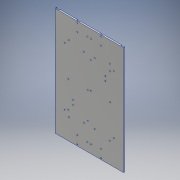
# Autodesk Inventor part: 밑판_수정
Saved by Autodesk Inventor 2017 (Build 210142000, 142)
## iProperties
Part Number: 밑판_수정
Material: 알루미늄 6061
Document SubType Name: Modeling
Designer: minom
Density: 2.7 g/cm^3
Appearance: 알루미늄 - 평지
Mass: 247.223 g
Surface Area: 1507.76 cm^2
Volume: 91.564 cm^3
Author: minom
Autodesk Inventor part; units mm, degrees
(part 1 of 2)
ref_plane "YZ Plane" through (0, 0, 0) normal (1, 0, 0) x (0, 1, 0)
ref_plane "XZ Plane" through (0, 0, 0) normal (0, 1, 0) x (-1, 0, 0)
ref_plane "XY Plane" through (0, 0, 0) normal (0, 0, 1) x (1, 0, 0)
sketch "스케치1" plane through (0, 0, 0) normal (0, 1, 0) x (-1, 0, 0)
  line L0 (0, 0) -> (-190, 0)
  line L1 (-190, 0) -> (-190, 300)
  line L2 (-190, 300) -> (0, 300)
  line L3 (0, 260) -> (0, 40)
  line L4 (0, 0) -> (40, 0)
  line L5 (40, 0) -> (40, 40)
  line L6 (40, 40) -> (0, 40)
  line L7 (0, 40) -> (0, 0)
  line L8 (-190, 0) -> (-230, 0)
  line L9 (-230, 0) -> (-230, 40)
  line L10 (-230, 40) -> (-190, 40)
  line L11 (-190, 40) -> (-190, 0)
  line L12 (-190, 300) -> (-230, 300)
  line L13 (-230, 300) -> (-230, 260)
  line L14 (-230, 260) -> (-190, 260)
  line L15 (-190, 260) -> (-190, 300)
  line L16 (0, 300) -> (40, 300)
  line L17 (40, 300) -> (40, 260)
  line L18 (40, 260) -> (0, 260)
  line L19 (0, 260) -> (0, 300)
  dimension "d0" = 190
  dimension "d1" = 300
  dimension "d2" = 40
  dimension "d3" = 40
  dimension "d4" = 40
  dimension "d5" = 40
  dimension "d6" = 40
  dimension "d7" = 40
  dimension "d8" = 40
  dimension "d9" = 40
  constraints: 40 end point, 10 parallel, 5 horizontal, 5 perpendicular
  measures "d0" distance of L1.end L2.end
  measures "d1" distance of L0.end L1.end
  measures "d2" distance of L3.end L5.end
  measures "d3" distance of L5.end L4.end
  measures "d4" distance of L9.end L10.end
  measures "d5" distance of L8.end L9.end
  measures "d6" distance of L14.end L13.end
  measures "d7" distance of L13.end L12.end
  measures "d8" distance of L3.start L17.end
  measures "d9" distance of L16.end L17.end
extrude "돌출1" add sketch "스케치1" along normal blind 4
sketch "스케치2" plane through (0, 4, 0) normal (0, 1, 0) x (1, 0, 0)
  line L0 (230, 0) -> (-40, 0) projected
  line L1 (-40, 0) -> (-40, -40) projected
  line L2 (-40, -40) -> (0, -40) projected
  line L3 (0, -40) -> (0, -260) projected
  line L4 (0, -260) -> (-40, -260) projected
  line L5 (-40, -260) -> (-40, -300) projected
  line L6 (-40, -300) -> (230, -300) projected
  line L7 (230, -300) -> (230, -260) projected
  line L8 (230, -260) -> (190, -260) projected
  line L9 (190, -260) -> (190, -40) projected
  line L10 (190, -40) -> (230, -40) projected
  line L11 (230, -40) -> (230, 0) projected
  line L12 (230, 0) -> (-40, 0) projected
  line L13 (-39, 0) -> (-30.8, 0)
  line L14 (-30.8, 0) -> (-30.8, -40)
  line L15 (-30.8, -40) -> (-39, -40)
  line L16 (-39, -40) -> (-39, 0)
  line L17 (-40, -300) -> (230, -300) projected
  line L18 (1, 0) -> (9.2, 0)
  line L19 (9.2, 0) -> (9.2, -300)
  line L20 (9.2, -300) -> (1, -300)
  line L21 (1, -300) -> (1, 0)
  line L22 (0, -260) -> (-40, -260) projected
  line L23 (-39, -260) -> (-30.8, -260)
  line L24 (-30.8, -260) -> (-30.8, -300)
  line L25 (-30.8, -300) -> (-39, -300)
  line L26 (-39, -300) -> (-39, -260)
  line L27 (190, -40) -> (230, -40) projected
  line L28 (229, 0) -> (220.8, 0)
  line L29 (220.8, 0) -> (220.8, -40)
  line L30 (220.8, -40) -> (229, -40)
  line L31 (229, -40) -> (229, 0)
  line L32 (189, 0) -> (180.8, 0)
  line L33 (180.8, 0) -> (180.8, -300)
  line L34 (180.8, -300) -> (189, -300)
  line L35 (189, -300) -> (189, 0)
  line L36 (229, -260) -> (220.8, -260)
  line L37 (220.8, -260) -> (220.8, -300)
  line L38 (220.8, -300) -> (229, -300)
  line L39 (229, -300) -> (229, -260)
  point P0 (0, 0)
  dimension "d12" = 8.2
  dimension "d13" = 8.2
  dimension "d14" = 8.2
  dimension "d15" = 8.2
  dimension "d16" = 1
  dimension "d17" = 1
  dimension "d18" = 1
  dimension "d19" = 1
  constraints: 48 end point, 16 point on line, 12 parallel, 6 horizontal, 6 perpendicular
  measures "d12" distance of L14.end L15.end
  measures "d13" distance of L19.end L20.end
  measures "d14" distance of L30.end L29.end
  measures "d15" distance of L34.end L33.end
  measures "d16" distance between parallel lines of L26 L5
  measures "d17" distance between parallel lines of L21 L3
  measures "d18" distance between parallel lines of L11 L31
  measures "d19" distance between parallel lines of L35 L9
extrude "돌출2" cut sketch "스케치2" against normal blind 2 contours L31 L10 L29 L0 | L35 L6 L33 L0 | L19 L6 L21 L0 | L37 L8 L39 L6 | L14 L2 L16 L0 | L6 L26 L4 L24
sketch "스케치4" plane through (0, 0, 0) normal (0, -1, 0) x (1, 0, 0)
  line L0 (220.8, 300) -> (220.8, 260) projected
  line L1 (220.8, 260) -> (190, 260) projected
  line L2 (190, 260) -> (190, 40) projected
  line L3 (190, 40) -> (220.8, 40) projected
  line L4 (220.8, 40) -> (220.8, 0) projected
  line L5 (220.8, 0) -> (189, 0) projected
  line L6 (189, 0) -> (189, 300) projected
  line L7 (189, 300) -> (220.8, 300) projected
  line L8 (9.2, 0) -> (9.2, 300) projected
  line L9 (9.2, 300) -> (180.8, 300) projected
  line L10 (180.8, 300) -> (180.8, 0) projected
  line L11 (180.8, 0) -> (9.2, 0) projected
  line L12 (1, 300) -> (1, 0) projected
  line L13 (1, 0) -> (-30.8, 0) projected
  line L14 (-30.8, 0) -> (-30.8, 40) projected
  line L15 (-30.8, 40) -> (0, 40) projected
  line L16 (0, 40) -> (0, 260) projected
  line L17 (0, 260) -> (-30.8, 260) projected
  line L18 (-30.8, 260) -> (-30.8, 300) projected
  line L19 (-30.8, 300) -> (1, 300) projected
  line L20 (214.8, 6) -> (194.8, 6)
  line L21 (193.8, 7) -> (193.8, 16)
  line L22 (194.8, 17) -> (214.8, 17)
  line L23 (215.8, 16) -> (215.8, 7)
  arc A0 (194.8, 17) -> (193.8, 16) centre (194.8, 16) ccw
  arc A1 (193.8, 7) -> (194.8, 6) centre (194.8, 7) ccw
  arc A2 (214.8, 6) -> (215.8, 7) centre (214.8, 7) ccw
  arc A3 (215.8, 16) -> (214.8, 17) centre (214.8, 16) ccw
  line L24 (194.8, 294) -> (214.8, 294)
  line L25 (215.8, 293) -> (215.8, 284)
  line L26 (214.8, 283) -> (194.8, 283)
  line L27 (193.8, 284) -> (193.8, 293)
  line L28 (-24.8, 294) -> (-4.8, 294)
  line L29 (-3.8, 293) -> (-3.8, 284)
  line L30 (-4.8, 283) -> (-24.8, 283)
  line L31 (-25.8, 284) -> (-25.8, 293)
  line L32 (-24.8, 17) -> (-4.8, 17)
  line L33 (-3.8, 16) -> (-3.8, 7)
  line L34 (-4.8, 6) -> (-24.8, 6)
  line L35 (-25.8, 7) -> (-25.8, 16)
  arc A4 (-24.8, 17) -> (-25.8, 16) centre (-24.8, 16) ccw
  arc A5 (-25.8, 7) -> (-24.8, 6) centre (-24.8, 7) ccw
  arc A6 (-4.8, 6) -> (-3.8, 7) centre (-4.8, 7) ccw
  arc A7 (-3.8, 16) -> (-4.8, 17) centre (-4.8, 16) ccw
  arc A8 (-25.8, 284) -> (-24.8, 283) centre (-24.8, 284) ccw
  arc A9 (-4.8, 283) -> (-3.8, 284) centre (-4.8, 284) ccw
  arc A10 (-3.8, 293) -> (-4.8, 294) centre (-4.8, 293) ccw
  arc A11 (-24.8, 294) -> (-25.8, 293) centre (-24.8, 293) ccw
  arc A12 (194.8, 294) -> (193.8, 293) centre (194.8, 293) ccw
  arc A13 (193.8, 284) -> (194.8, 283) centre (194.8, 284) ccw
  arc A14 (214.8, 283) -> (215.8, 284) centre (214.8, 284) ccw
  arc A15 (215.8, 293) -> (214.8, 294) centre (214.8, 293) ccw
  point P0 (0, 0)
  point P1 (215.8, 6)
  point P2 (193.8, 17)
  point P3 (193.8, 6)
  point P4 (215.8, 17)
  point P5 (215.8, 283)
  point P6 (215.8, 294)
  point P7 (193.8, 283)
  point P8 (-3.8, 283)
  point P9 (-3.8, 294)
  point P10 (-25.8, 283)
  point P11 (-3.8, 6)
  point P12 (-3.8, 17)
  point P13 (-25.8, 6)
  dimension "d24" = 22
  dimension "d25" = 11
  dimension "d26" = 5
  dimension "d27" = 23
  dimension "d30" = 1
  dimension "d31" = 22
  dimension "d32" = 11
  dimension "d33" = 5
  dimension "d34" = 23
  dimension "d35" = 22
  dimension "d36" = 11
  dimension "d37" = 5
  dimension "d38" = 23
  dimension "d39" = 22
  dimension "d40" = 11
  dimension "d41" = 5
  dimension "d42" = 23
  dimension "d43" = 1
  constraints: 32 end point, 32 point on circle, 32 tangent, 26 point on line, 16 centre point, 14 equal radius, 8 parallel, 4 horizontal, 4 perpendicular
  measures "d24" distance of point (193.8, 17) point (215.8, 17)
  measures "d25" distance of point (193.8, 6) point (193.8, 17)
  measures "d26" distance between parallel lines of L23 L4
  measures "d27" distance between parallel lines of L3 L22
  measures "d30" radius of A0
  measures "d31" distance of point (215.8, 283) point (193.8, 283)
  measures "d32" distance of point (215.8, 294) point (215.8, 283)
  measures "d33" distance between parallel lines of L25 L0
  measures "d34" distance between parallel lines of L1 L26
  measures "d35" distance of point (-3.8, 283) point (-25.8, 283)
  measures "d36" distance of point (-3.8, 294) point (-3.8, 283)
  measures "d37" distance between parallel lines of L31 L18
  measures "d38" distance between parallel lines of L30 L17
  measures "d39" distance of point (-3.8, 6) point (-25.8, 6)
  measures "d40" distance of point (-3.8, 17) point (-3.8, 6)
  measures "d41" distance between parallel lines of L35 L14
  measures "d42" distance between parallel lines of L32 L15
  measures "d43" radius of A4
extrude "돌출5" cut sketch "스케치4" against normal blind 10 contours L20 A1 L21 A0 L22 A3 L23 A2 | L24 A15 L25 A14 L26 A13 L27 A12 | L28 A10 L29 A9 L30 A8 L31 A11 | L32 A7 L33 A6 L34 A5 L35 A4
sketch "스케치5" plane through (0, 4, 0) normal (0, 1, 0) x (1, 0, 0)
  line L0 (9.2, 0) -> (9.2, -300) projected
  line L1 (9.2, -300) -> (180.8, -300) projected
  line L2 (180.8, -300) -> (180.8, 0) projected
  line L3 (180.8, 0) -> (9.2, 0) projected
  line L4 (135.8, -213.1) -> (144, -213.1)
  line L5 (144, -213.1) -> (144, -188.9)
  line L6 (144, -188.9) -> (135.8, -188.9)
  line L7 (135.8, -188.9) -> (135.8, -213.1)
  line L8 (190, -260) -> (190, -40) projected
  line L9 (46, -111.1) -> (54.2, -111.1)
  line L10 (54.2, -111.1) -> (54.2, -86.9)
  line L11 (54.2, -86.9) -> (46, -86.9)
  line L12 (46, -86.9) -> (46, -111.1)
  line L13 (0, -40) -> (0, -260) projected
  point P0 (0, 0)
  dimension "d46" = 8.2
  dimension "d47" = 24.2
  dimension "d48" = 86.9
  dimension "d49" = 46
  dimension "d50" = 8.2
  dimension "d51" = 24.2
  dimension "d52" = 86.9
  dimension "d53" = 46
  constraints: 16 end point, 4 parallel, 2 horizontal, 2 perpendicular
  measures "d46" distance of L6.end L5.end
  measures "d47" distance of L5.end L4.end
  measures "d48" distance between parallel lines of L4 L1
  measures "d49" distance between parallel lines of L8 L5
  measures "d50" distance of L11.end L10.end
  measures "d51" distance of L10.end L9.end
  measures "d52" distance between parallel lines of L3 L11
  measures "d53" distance between parallel lines of L13 L12
extrude "돌출6" cut sketch "스케치5" against normal blind 2 contours L7 L6 L5 L4 | L12 L11 L10 L9
sketch "스케치14" plane through (0, 4, 0) normal (0, 1, 0) x (1, 0, 0)
  line L0 (144, -188.9) -> (144, -213.1) projected
  line L1 (144, -213.1) -> (135.8, -213.1) projected
  line L2 (135.8, -213.1) -> (135.8, -188.9) projected
  line L3 (135.8, -188.9) -> (144, -188.9) projected
  line L4 (54.2, -86.9) -> (54.2, -111.1) projected
  line L5 (54.2, -111.1) -> (46, -111.1) projected
  line L6 (46, -111.1) -> (46, -86.9) projected
  line L7 (46, -86.9) -> (54.2, -86.9) projected
  line L8 (9.2, 0) -> (9.2, -300) projected
  line L9 (9.2, -300) -> (180.8, -300) projected
  line L10 (180.8, -300) -> (180.8, 0) projected
  line L11 (180.8, 0) -> (9.2, 0) projected
  line L12 (132, -300) -> (123.8, -300)
  line L13 (123.8, -300) -> (123.8, -260)
  line L14 (123.8, -260) -> (132, -260)
  line L15 (132, -260) -> (132, -300)
  line L16 (230, -300) -> (230, -260) projected
  line L17 (-40, -300) -> (230, -300) projected
  line L18 (66.2, -300) -> (58, -300)
  line L19 (58, -300) -> (58, -260)
  line L20 (58, -260) -> (66.2, -260)
  line L21 (66.2, -260) -> (66.2, -300)
  line L22 (-40, -260) -> (-40, -300) projected
  line L23 (58, 0) -> (66.2, 0)
  line L24 (66.2, 0) -> (66.2, -40)
  line L25 (66.2, -40) -> (58, -40)
  line L26 (58, -40) -> (58, 0)
  line L27 (123.8, 0) -> (132, 0)
  line L28 (132, 0) -> (132, -40)
  line L29 (132, -40) -> (123.8, -40)
  line L30 (123.8, -40) -> (123.8, 0)
  line L31 (230, -40) -> (230, 0) projected
  line L32 (-40, 0) -> (-40, -40) projected
  line L33 (189, 0) -> (189, -300) projected
  line L34 (190, -260) -> (190, -40) projected
  line L35 (190, -40) -> (220.8, -40) projected
  line L36 (220.8, -40) -> (220.8, 0) projected
  line L37 (220.8, 0) -> (189, 0) projected
  line L38 (189, -300) -> (220.8, -300) projected
  line L39 (220.8, -300) -> (220.8, -260) projected
  line L40 (220.8, -260) -> (190, -260) projected
  point P0 (0, 0)
  dimension "d184" = 8.2
  dimension "d185" = 40
  dimension "d186" = 98
  dimension "d187" = 8.2
  dimension "d188" = 40
  dimension "d189" = 98
  dimension "d190" = 8.2
  dimension "d191" = 40
  dimension "d192" = 8.2
  dimension "d193" = 40
  dimension "d194" = 98
  dimension "d195" = 98
  constraints: 32 end point, 8 parallel, 4 horizontal, 4 perpendicular, 4 point on line
  measures "d184" distance of L13.end L14.end
  measures "d185" distance of L12.end L13.end
  measures "d186" distance between parallel lines of L15 L16
  measures "d187" distance of L19.end L20.end
  measures "d188" distance of L18.end L19.end
  measures "d189" distance between parallel lines of L22 L19
  measures "d190" distance of L24.end L25.end
  measures "d191" distance of L23.end L24.end
  measures "d192" distance of L28.end L29.end
  measures "d193" distance of L27.end L28.end
  measures "d194" distance between parallel lines of L28 L31
  measures "d195" distance between parallel lines of L26 L32
extrude "돌출14" cut sketch "스케치14" against normal blind 2 contours L11 L24 L25 L26 | L19 L20 L21 L9 | L11 L28 L29 L30 | L13 L14 L15 L9
sketch "스케치22" plane through (0, 0, 0) normal (0, -1, 0) x (1, 0, 0)
  arc A0 (-35.9607, 3.3386) -> (-33.8393, 3.3386) centre (-34.9, 4) ccw projected
  arc A1 (-33.8393, 4.6614) -> (-35.9607, 4.6614) centre (-34.9, 4) ccw projected
  ellipse E0 centre (-34.9, 5.617) end of major axis (-34.9, 7.0604) minor radius 1.25 (-36.0761, 5.1282) -> (-35.9985, 4.9282) ccw projected
  line L0 (-35.9985, 4.9282) -> (-37.9, 4.9282) projected
  line L1 (-37.9, 4.9282) -> (-37.9, 42) projected
  line L2 (-30.9, 42) -> (-37.9, 42) projected
  line L3 (-30.9, 4.9282) -> (-30.9, 42) projected
  line L4 (-30.9, 4.9282) -> (-33.8015, 4.9282) projected
  ellipse E1 centre (-34.9, 5.617) end of major axis (-34.9, 7.0604) minor radius 1.25 (-33.8015, 4.9282) -> (-33.7239, 5.1282) ccw projected
  line L5 (-33.7239, 5.1282) -> (-34.3618, 5.1282) projected
  arc A2 (-34.3618, 5.1282) -> (-35.4382, 5.1282) centre (-34.9, 4) ccw projected
  line L6 (-35.4382, 5.1282) -> (-36.0761, 5.1282) projected
  circle A3 centre (-34.9, 26) radius 1.25 projected
  circle A4 centre (62.1, 25.9714) radius 1.25 projected
  line L7 (61.6263, 5.1282) -> (61.2311, 5.1282) projected
  ellipse E2 centre (62.1, 6.1658) end of major axis (62.1, 7.6092) minor radius 1.25 (61.2311, 5.1282) -> (61.3752, 4.9898) ccw projected
  arc A5 (61.3752, 4.9898) -> (61.2956, 4.9282) centre (62.1, 3.9714) ccw projected
  line L8 (58.1, 4.9282) -> (61.2956, 4.9282) projected
  line L9 (58.1, 36) -> (58.1, 4.9282) projected
  line L10 (58.1, 36) -> (66.1, 36) projected
  line L11 (66.1, 4.9282) -> (66.1, 36) projected
  line L12 (62.9044, 4.9282) -> (66.1, 4.9282) projected
  arc A6 (62.9044, 4.9282) -> (62.8248, 4.9898) centre (62.1, 3.9714) ccw projected
  ellipse E3 centre (62.1, 6.1658) end of major axis (62.1, 7.6092) minor radius 1.25 (62.8248, 4.9898) -> (62.9689, 5.1282) ccw projected
  line L13 (62.9689, 5.1282) -> (62.5737, 5.1282) projected
  arc A7 (62.5737, 5.1282) -> (61.6263, 5.1282) centre (62.1, 3.9714) ccw projected
  circle A8 centre (127.9, 25.9714) radius 1.25 projected
  line L14 (127.4263, 5.1282) -> (127.0311, 5.1282) projected
  ellipse E4 centre (127.9, 6.1658) end of major axis (127.9, 7.6092) minor radius 1.25 (127.0311, 5.1282) -> (127.1752, 4.9898) ccw projected
  arc A9 (127.1752, 4.9898) -> (127.0956, 4.9282) centre (127.9, 3.9714) ccw projected
  line L15 (123.9, 4.9282) -> (127.0956, 4.9282) projected
  line L16 (123.9, 36) -> (123.9, 4.9282) projected
  line L17 (123.9, 36) -> (131.9, 36) projected
  line L18 (131.9, 4.9282) -> (131.9, 36) projected
  line L19 (128.7044, 4.9282) -> (131.9, 4.9282) projected
  arc A10 (128.7044, 4.9282) -> (128.6248, 4.9898) centre (127.9, 3.9714) ccw projected
  ellipse E5 centre (127.9, 6.1658) end of major axis (127.9, 7.6092) minor radius 1.25 (128.6248, 4.9898) -> (128.7689, 5.1282) ccw projected
  line L20 (128.7689, 5.1282) -> (128.3737, 5.1282) projected
  arc A11 (128.3737, 5.1282) -> (127.4263, 5.1282) centre (127.9, 3.9714) ccw projected
  line L21 (226.0761, 5.1282) -> (225.4382, 5.1282) projected
  arc A12 (225.4382, 5.1282) -> (224.3618, 5.1282) centre (224.9, 4) ccw projected
  line L22 (224.3618, 5.1282) -> (223.7239, 5.1282) projected
  ellipse E6 centre (224.9, 5.617) end of major axis (224.9, 7.0604) minor radius 1.25 (223.7239, 5.1282) -> (223.8015, 4.9282) ccw projected
  line L23 (220.9, 4.9282) -> (223.8015, 4.9282) projected
  line L24 (220.9, 42) -> (220.9, 4.9282) projected
  line L25 (220.9, 42) -> (227.9, 42) projected
  line L26 (227.9, 42) -> (227.9, 4.9282) projected
  line L27 (225.9985, 4.9282) -> (227.9, 4.9282) projected
  ellipse E7 centre (224.9, 5.617) end of major axis (224.9, 7.0604) minor radius 1.25 (225.9985, 4.9282) -> (226.0761, 5.1282) ccw projected
  circle A13 centre (224.9, 26) radius 1.25 projected
  ellipse E8 centre (224.9, 294.383) end of major axis (224.9, 292.9396) minor radius 1.25 (226.0761, 294.8718) -> (225.9985, 295.0718) ccw projected
  line L28 (225.9985, 295.0718) -> (227.9, 295.0718) projected
  line L29 (227.9, 295.0718) -> (227.9, 258) projected
  line L30 (220.9, 258) -> (227.9, 258) projected
  line L31 (220.9, 295.0718) -> (220.9, 258) projected
  line L32 (220.9, 295.0718) -> (223.8015, 295.0718) projected
  ellipse E9 centre (224.9, 294.383) end of major axis (224.9, 292.9396) minor radius 1.25 (223.8015, 295.0718) -> (223.7239, 294.8718) ccw projected
  line L33 (223.7239, 294.8718) -> (224.3618, 294.8718) projected
  arc A14 (224.3618, 294.8718) -> (225.4382, 294.8718) centre (224.9, 296) ccw projected
  line L34 (225.4382, 294.8718) -> (226.0761, 294.8718) projected
  circle A15 centre (224.9, 274) radius 1.25 projected
  circle A16 centre (127.9, 274.0286) radius 1.25 projected
  line L35 (128.3737, 294.8718) -> (128.7689, 294.8718) projected
  ellipse E10 centre (127.9, 293.8342) end of major axis (127.9, 292.3908) minor radius 1.25 (128.7689, 294.8718) -> (128.6248, 295.0102) ccw projected
  arc A17 (128.6248, 295.0102) -> (128.7044, 295.0718) centre (127.9, 296.0286) ccw projected
  line L36 (131.9, 295.0718) -> (128.7044, 295.0718) projected
  line L37 (131.9, 264) -> (131.9, 295.0718) projected
  line L38 (131.9, 264) -> (123.9, 264) projected
  line L39 (123.9, 295.0718) -> (123.9, 264) projected
  line L40 (127.0956, 295.0718) -> (123.9, 295.0718) projected
  arc A18 (127.0956, 295.0718) -> (127.1752, 295.0102) centre (127.9, 296.0286) ccw projected
  ellipse E11 centre (127.9, 293.8342) end of major axis (127.9, 292.3908) minor radius 1.25 (127.1752, 295.0102) -> (127.0311, 294.8718) ccw projected
  line L41 (127.0311, 294.8718) -> (127.4263, 294.8718) projected
  arc A19 (127.4263, 294.8718) -> (128.3737, 294.8718) centre (127.9, 296.0286) ccw projected
  circle A20 centre (62.1, 274.0286) radius 1.25 projected
  line L42 (62.5737, 294.8718) -> (62.9689, 294.8718) projected
  ellipse E12 centre (62.1, 293.8342) end of major axis (62.1, 292.3908) minor radius 1.25 (62.9689, 294.8718) -> (62.8248, 295.0102) ccw projected
  arc A21 (62.8248, 295.0102) -> (62.9044, 295.0718) centre (62.1, 296.0286) ccw projected
  line L43 (66.1, 295.0718) -> (62.9044, 295.0718) projected
  line L44 (66.1, 264) -> (66.1, 295.0718) projected
  line L45 (66.1, 264) -> (58.1, 264) projected
  line L46 (58.1, 295.0718) -> (58.1, 264) projected
  line L47 (61.2956, 295.0718) -> (58.1, 295.0718) projected
  arc A22 (61.2956, 295.0718) -> (61.3752, 295.0102) centre (62.1, 296.0286) ccw projected
  ellipse E13 centre (62.1, 293.8342) end of major axis (62.1, 292.3908) minor radius 1.25 (61.3752, 295.0102) -> (61.2311, 294.8718) ccw projected
  line L48 (61.2311, 294.8718) -> (61.6263, 294.8718) projected
  arc A23 (61.6263, 294.8718) -> (62.5737, 294.8718) centre (62.1, 296.0286) ccw projected
  line L49 (-36.0761, 294.8718) -> (-35.4382, 294.8718) projected
  arc A24 (-35.4382, 294.8718) -> (-34.3618, 294.8718) centre (-34.9, 296) ccw projected
  line L50 (-34.3618, 294.8718) -> (-33.7239, 294.8718) projected
  ellipse E14 centre (-34.9, 294.383) end of major axis (-34.9, 292.9396) minor radius 1.25 (-33.7239, 294.8718) -> (-33.8015, 295.0718) ccw projected
  line L51 (-30.9, 295.0718) -> (-33.8015, 295.0718) projected
  line L52 (-30.9, 258) -> (-30.9, 295.0718) projected
  line L53 (-30.9, 258) -> (-37.9, 258) projected
  line L54 (-37.9, 258) -> (-37.9, 295.0718) projected
  line L55 (-35.9985, 295.0718) -> (-37.9, 295.0718) projected
  ellipse E15 centre (-34.9, 294.383) end of major axis (-34.9, 292.9396) minor radius 1.25 (-35.9985, 295.0718) -> (-36.0761, 294.8718) ccw projected
  circle A25 centre (-34.9, 274) radius 1.25 projected
  circle A26 centre (127.9, 3.9714) radius 1.5
  circle A27 centre (224.9, 4) radius 1.5
  circle A28 centre (62.1, 3.9714) radius 1.5
  circle A29 centre (62.1, 25.9714) radius 1.5
  circle A30 centre (-34.9, 26) radius 1.5
  circle A31 centre (-34.9, 4) radius 1.5
  circle A32 centre (127.9, 25.9714) radius 1.5
  circle A33 centre (224.9, 26) radius 1.5
  circle A34 centre (224.9, 274) radius 1.5
  circle A35 centre (224.9, 296) radius 1.5
  circle A36 centre (127.9, 274.0286) radius 1.5
  circle A37 centre (127.9, 296.0286) radius 1.5
  circle A38 centre (62.1, 274.0286) radius 1.5
  circle A39 centre (62.1, 296.0286) radius 1.5
  circle A40 centre (-34.9, 274) radius 1.5
  circle A41 centre (-34.9, 296) radius 1.5
  point P0 (0, 0)
  dimension "d416" = 3
  dimension "d417" = 3
  dimension "d418" = 3
  dimension "d419" = 3
  dimension "d420" = 3
  dimension "d421" = 3
  dimension "d422" = 3
  dimension "d423" = 3
  dimension "d424" = 3
  dimension "d425" = 3
  dimension "d426" = 3
  dimension "d427" = 3
  dimension "d428" = 3
  dimension "d429" = 3
  dimension "d430" = 3
  dimension "d431" = 3
  constraints: 16 centre point, 16 coincident, 16 other
  measures "d416" diameter of A26
  measures "d417" diameter of A27
  measures "d418" diameter of A28
  measures "d419" diameter of A29
  measures "d420" diameter of A30
  measures "d421" diameter of A31
  measures "d422" diameter of A32
  measures "d423" diameter of A33
  measures "d424" diameter of A34
  measures "d425" diameter of A35
  measures "d426" diameter of A36
  measures "d427" diameter of A37
  measures "d428" diameter of A38
  measures "d429" diameter of A39
  measures "d430" diameter of A40
  measures "d431" diameter of A41
extrude "돌출21" cut sketch "스케치22" against normal blind 2 contours L5 A31 E1 L4 L0 E0 L6 A1 | A1 L6 A31 L5 | A31 L4 E1 | E0 L0 A31 | A3 | A4 | A7 L13 E3 A6 L12 A28 L8 A5 E2 L7 | L7 E2 A5 L8 A28 L12 A6 E3 L13 A7 | A8 | A11 L20 E5 A10 L19 A26 L15 A9 E4 L14 | L14 E4 A9 L15 A26 L19 A10 E5 L20 A11 | A27 E7 L27 L23 E6 L22 A12 L21 | L21 A12 L22 A27 | A27 L27 E7 | E6 L23 A27 | A13 | A35 L34 A14 L33 E9 L32 L28 E8 | E8 L28 A35 | A35 L33 A14 L34 | A35 L32 E9 | A15 | A16 | A19 L41 E11 A18 L40 A37 L36 A17 E10 L35 | L35 E10 A17 L36 A37 L40 A18 E11 L41 A19 | A20 | A23 L48 E13 A22 L47 A39 L43 A21 E12 L42 | L42 E12 A21 L43 A39 L47 A22 E13 L48 A23 | A41 E15 L55 L51 E14 L50 A24 L49 | L49 A24 L50 A41 | A41 L55 E15 | E14 L51 A41 | A25 | A29 | A30 | A32 | A33 | A34 | A36 | A38 | A40
sketch "스케치23" plane through (0, 2, 0) normal (0, 1, 0) x (1, 0, 0)
  circle A0 centre (50.1, -93) radius 1.25 projected
  circle A1 centre (50.1, -105) radius 1.25 projected
  line L0 (46.1, -107) -> (46.1, -91) projected
  line L1 (46.1, -107) -> (54.1, -107) projected
  line L2 (54.1, -91) -> (54.1, -107) projected
  line L3 (46.1, -91) -> (54.1, -91) projected
  circle A2 centre (139.9, -207) radius 1.25 projected
  circle A3 centre (139.9, -195) radius 1.25 projected
  line L4 (143.9, -193) -> (143.9, -209) projected
  line L5 (143.9, -193) -> (135.9, -193) projected
  line L6 (135.9, -209) -> (135.9, -193) projected
  line L7 (143.9, -209) -> (135.9, -209) projected
  circle A4 centre (139.9, -207) radius 1.5
  circle A5 centre (139.9, -195) radius 1.5
  circle A6 centre (50.1, -105) radius 1.5
  circle A7 centre (50.1, -93) radius 1.5
  point P0 (0, 0)
  dimension "d434" = 3
  dimension "d435" = 3
  dimension "d436" = 3
  dimension "d437" = 3
  constraints: 4 centre point, 4 coincident
  measures "d434" diameter of A4
  measures "d435" diameter of A5
  measures "d436" diameter of A6
  measures "d437" diameter of A7
extrude "돌출22" cut sketch "스케치23" against normal blind 2 contours A0 | A1 | A2 | A3 | A4 | A5 | A6 | A7
sketch "스케치24" plane through (0, 4, 0) normal (0, 1, 0) x (1, 0, 0)
  line L0 (58, -40) -> (58, 0) projected
  line L1 (58, 0) -> (9.2, 0) projected
  line L2 (9.2, 0) -> (9.2, -300) projected
  line L3 (9.2, -300) -> (58, -300) projected
  line L4 (58, -300) -> (58, -260) projected
  line L5 (58, -260) -> (66.2, -260) projected
  line L6 (66.2, -260) -> (66.2, -300) projected
  line L7 (66.2, -300) -> (123.8, -300) projected
  line L8 (123.8, -300) -> (123.8, -260) projected
  line L9 (123.8, -260) -> (132, -260) projected
  line L10 (132, -260) -> (132, -300) projected
  line L11 (132, -300) -> (180.8, -300) projected
  line L12 (180.8, -300) -> (180.8, 0) projected
  line L13 (180.8, 0) -> (132, 0) projected
  line L14 (132, 0) -> (132, -40) projected
  line L15 (132, -40) -> (123.8, -40) projected
  line L16 (123.8, -40) -> (123.8, 0) projected
  line L17 (123.8, 0) -> (66.2, 0) projected
  line L18 (66.2, 0) -> (66.2, -40) projected
  line L19 (66.2, -40) -> (58, -40) projected
  line L20 (144, -188.9) -> (144, -213.1) projected
  line L21 (144, -213.1) -> (135.8, -213.1) projected
  line L22 (135.8, -213.1) -> (135.8, -188.9) projected
  line L23 (135.8, -188.9) -> (144, -188.9) projected
  line L24 (54.2, -86.9) -> (54.2, -111.1) projected
  line L25 (54.2, -111.1) -> (46, -111.1) projected
  line L26 (46, -111.1) -> (46, -86.9) projected
  line L27 (46, -86.9) -> (54.2, -86.9) projected
  circle A0 centre (132, -260) radius 1.5
  circle A1 centre (123.8, -260) radius 1.5
  line L28 (66.2, -260) -> (66.2, -300) projected
  circle A2 centre (66.2, -260) radius 1.5
  circle A3 centre (58, -260) radius 1.5
  line L29 (144, -213.1) -> (135.8, -213.1) projected
  circle A4 centre (135.8, -213.1) radius 1.5
  circle A5 centre (144, -213.1) radius 1.5
  circle A6 centre (144, -188.9) radius 1.5
  circle A7 centre (135.8, -188.9) radius 1.5
  circle A8 centre (46, -111.1) radius 1.5
  line L30 (54.2, -111.1) -> (46, -111.1) projected
  circle A9 centre (54.2, -111.1) radius 1.5
  line L31 (54.2, -86.9) -> (54.2, -111.1) projected
  circle A10 centre (54.2, -86.9) radius 1.5
  circle A11 centre (46, -86.9) radius 1.5
  circle A12 centre (58, -40) radius 1.5
  line L32 (66.2, -40) -> (58, -40) projected
  circle A13 centre (66.2, -40) radius 1.5
  line L33 (132, -40) -> (123.8, -40) projected
  circle A14 centre (123.8, -40) radius 1.5
  circle A15 centre (132, -40) radius 1.5
  point P0 (0, 0)
  dimension "d440" = 3
  dimension "d441" = 3
  dimension "d442" = 3
  dimension "d443" = 3
  dimension "d444" = 3
  dimension "d445" = 3
  dimension "d446" = 3
  dimension "d447" = 3
  dimension "d448" = 3
  dimension "d449" = 3
  dimension "d450" = 3
  dimension "d451" = 3
  dimension "d452" = 3
  dimension "d453" = 3
  dimension "d454" = 3
  dimension "d455" = 3
  constraints: 16 centre point, 16 coincident
  measures "d440" diameter of A0
  measures "d441" diameter of A1
  measures "d442" diameter of A2
  measures "d443" diameter of A3
  measures "d444" diameter of A4
  measures "d445" diameter of A5
  measures "d446" diameter of A6
  measures "d447" diameter of A7
  measures "d448" diameter of A8
  measures "d449" diameter of A9
  measures "d450" diameter of A10
  measures "d451" diameter of A11
  measures "d452" diameter of A12
  measures "d453" diameter of A13
  measures "d454" diameter of A14
  measures "d455" diameter of A15
extrude "돌출23" cut sketch "스케치24" against normal blind 2 contours L19 A12 L0 | L0 A12 L19 | A13 L18 L19 | L19 L18 A13 | A3 L5 L4 | L4 L5 A3 | A14 L15 L16 | L16 L15 A14 | A2 L6 L5 | L5 L6 A2 | A15 L14 L15 | L15 L14 A15 | A1 L9 L8 | L8 L9 A1 | A0 L10 L9 | L9 L10 A0 | L23 A6 L20 | L20 A6 L23 | A5 L21 L20 | L20 L21 A5 | A7 L22 L23 | L23 L22 A7 | A4 L22 L21 | L21 L22 A4 | L27 A10 L24 | L24 A10 L27 | A9 L25 L24 | L24 L25 A9 | A11 L26 L27 | L27 L26 A11 | A8 L26 L25 | L25 L26 A8
sketch "스케치25" plane through (0, 4, 0) normal (0, 1, 0) x (1, 0, 0)
  arc A0 (132.9, -148) -> (137.9, -153) centre (132.9, -153) ccw projected
  line L0 (132.9, -148) -> (95.9, -148) projected
  line L1 (95.9, -148) -> (95.9, -228) projected
  line L2 (95.9, -228) -> (127.9, -228) projected
  circle A1 centre (127.9, -223) radius 5 projected
  line L3 (127.9, -228) -> (155.9, -228) projected
  line L4 (155.9, -228) -> (155.9, -148) projected
  line L5 (155.9, -148) -> (142.9, -148) projected
  arc A2 (137.9, -153) -> (142.9, -148) centre (142.9, -153) ccw projected
  circle A3 centre (98.9, -225) radius 1.5 projected
  circle A4 centre (152.9, -151) radius 1.5 projected
  circle A5 centre (152.9, -225) radius 1.5 projected
  circle A6 centre (98.9, -151) radius 1.5 projected
  arc A7 (57.1, -152) -> (52.1, -147) centre (57.1, -147) ccw projected
  line L6 (57.1, -152) -> (94.1, -152) projected
  line L7 (94.1, -152) -> (94.1, -72) projected
  line L8 (94.1, -72) -> (62.1, -72) projected
  circle A8 centre (62.1, -77) radius 5 projected
  line L9 (62.1, -72) -> (34.1, -72) projected
  line L10 (34.1, -72) -> (34.1, -152) projected
  line L11 (34.1, -152) -> (47.1, -152) projected
  arc A9 (52.1, -147) -> (47.1, -152) centre (47.1, -147) ccw projected
  circle A10 centre (91.1, -75) radius 1.5 projected
  circle A11 centre (37.1, -149) radius 1.5 projected
  circle A12 centre (37.1, -75) radius 1.5 projected
  circle A13 centre (91.1, -149) radius 1.5 projected
  point P0 (0, 0)
extrude "돌출24" cut sketch "스케치25" against normal blind 4 contours A3 | A4 | A5 | A6 | A10 | A11 | A12 | A13
sketch "스케치26" plane through (0, 4, 0) normal (0, 1, 0) x (1, 0, 0)
  line L0 (-19.9, -32) -> (-19.9, -27) projected
  line L1 (-19.9, -27) -> (-9.9, -27) projected
  line L2 (-9.9, -27) -> (-9.9, -32) projected
  line L3 (-9.9, -32) -> (-19.9, -32) projected
  circle A0 centre (-9.9, -23) radius 1.5 projected
  circle A1 centre (-19.9, -23) radius 1.5 projected
  line L4 (-24.9, -34) -> (-4.9, -34) projected
  line L5 (-4.9, -34) -> (-4.9, -7) projected
  line L6 (-4.9, -7) -> (-24.9, -7) projected
  line L7 (-24.9, -7) -> (-24.9, -34) projected
  line L8 (199.9, -32) -> (199.9, -27) projected
  line L9 (199.9, -27) -> (209.9, -27) projected
  line L10 (209.9, -27) -> (209.9, -32) projected
  line L11 (209.9, -32) -> (199.9, -32) projected
  circle A2 centre (209.9, -23) radius 1.5 projected
  circle A3 centre (199.9, -23) radius 1.5 projected
  line L12 (194.9, -34) -> (214.9, -34) projected
  line L13 (214.9, -34) -> (214.9, -7) projected
  line L14 (214.9, -7) -> (194.9, -7) projected
  line L15 (194.9, -7) -> (194.9, -34) projected
  line L16 (209.9, -268) -> (209.9, -273) projected
  line L17 (209.9, -273) -> (199.9, -273) projected
  line L18 (199.9, -273) -> (199.9, -268) projected
  line L19 (199.9, -268) -> (209.9, -268) projected
  circle A4 centre (199.9, -277) radius 1.5 projected
  circle A5 centre (209.9, -277) radius 1.5 projected
  line L20 (214.9, -266) -> (194.9, -266) projected
  line L21 (194.9, -266) -> (194.9, -293) projected
  line L22 (194.9, -293) -> (214.9, -293) projected
  line L23 (214.9, -293) -> (214.9, -266) projected
  line L24 (-9.9, -268) -> (-9.9, -273) projected
  line L25 (-9.9, -273) -> (-19.9, -273) projected
  line L26 (-19.9, -273) -> (-19.9, -268) projected
  line L27 (-19.9, -268) -> (-9.9, -268) projected
  circle A6 centre (-19.9, -277) radius 1.5 projected
  circle A7 centre (-9.9, -277) radius 1.5 projected
  line L28 (-4.9, -266) -> (-24.9, -266) projected
  line L29 (-24.9, -266) -> (-24.9, -293) projected
  line L30 (-24.9, -293) -> (-4.9, -293) projected
  line L31 (-4.9, -293) -> (-4.9, -266) projected
  point P0 (0, 0)
extrude "돌출25" cut sketch "스케치26" against normal blind 4 contours A0 | A1 | A2 | A3 | A4 | A5 | A6 | A7
sketch "스케치27" plane through (0, 4, 0) normal (0, 1, 0) x (1, 0, 0)
  circle A0 centre (38.5558, -57.435) radius 1.25 projected
  circle A1 centre (26.535, -69.4558) radius 1.25 projected
  circle A2 centre (151.4442, -57.435) radius 1.25 projected
  circle A3 centre (163.465, -69.4558) radius 1.25 projected
  circle A4 centre (110.0091, -65) radius 1.25 projected
  circle A5 centre (80.0091, -65) radius 1.25 projected
  circle A6 centre (80.0091, -235) radius 1.25 projected
  circle A7 centre (110.0091, -235) radius 1.25 projected
  circle A8 centre (38.5558, -242.565) radius 1.25 projected
  circle A9 centre (26.535, -230.5442) radius 1.25 projected
  circle A10 centre (151.4442, -242.565) radius 1.25 projected
  circle A11 centre (163.465, -230.5442) radius 1.25 projected
  circle A12 centre (163.465, -230.5442) radius 1.5
  circle A13 centre (151.4442, -242.565) radius 1.5
  circle A14 centre (110.0091, -235) radius 1.5
  circle A15 centre (80.0091, -235) radius 1.5
  circle A16 centre (38.5558, -242.565) radius 1.5
  circle A17 centre (26.535, -230.5442) radius 1.5
  circle A18 centre (26.535, -69.4558) radius 1.5
  circle A19 centre (38.5558, -57.435) radius 1.5
  circle A20 centre (80.0091, -65) radius 1.5
  circle A21 centre (110.0091, -65) radius 1.5
  circle A22 centre (151.4442, -57.435) radius 1.5
  circle A23 centre (163.465, -69.4558) radius 1.5
  point P0 (0, 0)
  dimension "d462" = 3
  dimension "d463" = 3
  dimension "d464" = 3
  dimension "d465" = 3
  dimension "d466" = 3
  dimension "d467" = 3
  dimension "d468" = 3
  dimension "d469" = 3
  dimension "d470" = 3
  dimension "d471" = 3
  dimension "d472" = 3
  dimension "d473" = 3
  constraints: 12 centre point, 1 coincident
  measures "d462" diameter of A12
  measures "d463" diameter of A13
  measures "d464" diameter of A14
  measures "d465" diameter of A15
  measures "d466" diameter of A16
  measures "d467" diameter of A17
  measures "d468" diameter of A18
  measures "d469" diameter of A19
  measures "d470" diameter of A20
  measures "d471" diameter of A21
  measures "d472" diameter of A22
  measures "d473" diameter of A23
extrude "돌출26" cut sketch "스케치27" against normal blind 4 contours A0 | A1 | A2 | A3 | A4 | A5 | A6 | A7 | A8 | A9 | A10 | A11 | A12 | A13 | A14 | A15 | A16 | A17 | A18 | A19 | A20 | A21 | A22 | A23
sketch "스케치28" plane through (0, 4, 0) normal (0, 1, 0) x (1, 0, 0)
  circle A0 centre (100, -23) radius 1.5 projected
  circle A1 centre (90, -23) radius 1.5 projected
  circle A2 centre (95, -15) radius 2.5 projected
  line L0 (100, -27) -> (100, -32) projected
  line L1 (100, -32) -> (90, -32) projected
  line L2 (90, -32) -> (90, -27) projected
  line L3 (90, -27) -> (100, -27) projected
  line L4 (105, -7) -> (85, -7) projected
  line L5 (85, -7) -> (85, -34) projected
  line L6 (85, -34) -> (105, -34) projected
  line L7 (105, -34) -> (105, -7) projected
  circle A3 centre (90, -277) radius 1.5 projected
  circle A4 centre (100, -277) radius 1.5 projected
  circle A5 centre (95, -285) radius 2.5 projected
  line L8 (90, -273) -> (90, -268) projected
  line L9 (90, -268) -> (100, -268) projected
  line L10 (100, -268) -> (100, -273) projected
  line L11 (100, -273) -> (90, -273) projected
  line L12 (85, -293) -> (105, -293) projected
  line L13 (105, -293) -> (105, -266) projected
  line L14 (105, -266) -> (85, -266) projected
  line L15 (85, -266) -> (85, -293) projected
  point P0 (0, 0)
extrude "돌출27" cut sketch "스케치28" against normal blind 4 contours A0 | A1 | A3 | A4
sketch "스케치29" plane through (0, 4, 0) normal (0, 1, 0) x (1, 0, 0)
  circle A0 centre (90, -277) radius 1.5 projected
  circle A1 centre (100, -23) radius 1.5 projected
  circle A2 centre (90, -23) radius 1.5 projected
  circle A3 centre (100, -277) radius 1.5 projected
  circle A4 centre (151.4442, -57.435) radius 1.5 projected
  circle A5 centre (80.0091, -65) radius 1.5 projected
  circle A6 centre (26.535, -69.4558) radius 1.5 projected
  circle A7 centre (38.5558, -242.565) radius 1.5 projected
  circle A8 centre (110.0091, -235) radius 1.5 projected
  circle A9 centre (163.465, -230.5442) radius 1.5 projected
  circle A10 centre (151.4442, -242.565) radius 1.5 projected
  circle A11 centre (80.0091, -235) radius 1.5 projected
  circle A12 centre (26.535, -230.5442) radius 1.5 projected
  circle A13 centre (38.5558, -57.435) radius 1.5 projected
  circle A14 centre (110.0091, -65) radius 1.5 projected
  circle A15 centre (163.465, -69.4558) radius 1.5 projected
  circle A16 centre (37.1, -75) radius 1.5 projected
  circle A17 centre (91.1, -75) radius 1.5 projected
  circle A18 centre (152.9, -225) radius 1.5 projected
  circle A19 centre (98.9, -225) radius 1.5 projected
  circle A20 centre (152.9, -151) radius 1.5 projected
  circle A21 centre (98.9, -151) radius 1.5 projected
  circle A22 centre (37.1, -149) radius 1.5 projected
  circle A23 centre (91.1, -149) radius 1.5 projected
  arc A24 (47.5, -86.9) -> (46, -88.4) centre (46, -86.9) ccw projected
  line L0 (47.5, -86.9) -> (52.7, -86.9) projected
  arc A25 (54.2, -88.4) -> (52.7, -86.9) centre (54.2, -86.9) ccw projected
  line L1 (54.2, -88.4) -> (54.2, -109.6) projected
  arc A26 (52.7, -111.1) -> (54.2, -109.6) centre (54.2, -111.1) ccw projected
  line L2 (52.7, -111.1) -> (47.5, -111.1) projected
  arc A27 (46, -109.6) -> (47.5, -111.1) centre (46, -111.1) ccw projected
  line L3 (46, -109.6) -> (46, -88.4) projected
  arc A28 (137.3, -188.9) -> (135.8, -190.4) centre (135.8, -188.9) ccw projected
  line L4 (137.3, -188.9) -> (142.5, -188.9) projected
  arc A29 (144, -190.4) -> (142.5, -188.9) centre (144, -188.9) ccw projected
  line L5 (144, -190.4) -> (144, -211.6) projected
  arc A30 (142.5, -213.1) -> (144, -211.6) centre (144, -213.1) ccw projected
  line L6 (142.5, -213.1) -> (137.3, -213.1) projected
  arc A31 (135.8, -211.6) -> (137.3, -213.1) centre (135.8, -213.1) ccw projected
  line L7 (135.8, -211.6) -> (135.8, -190.4) projected
  arc A32 (130.5, -40) -> (132, -38.5) centre (132, -40) ccw projected
  line L8 (130.5, -40) -> (125.3, -40) projected
  arc A33 (123.8, -38.5) -> (125.3, -40) centre (123.8, -40) ccw projected
  line L9 (123.8, -38.5) -> (123.8, 0) projected
  line L10 (123.8, 0) -> (66.2, 0) projected
  line L11 (66.2, 0) -> (66.2, -38.5) projected
  arc A34 (64.7, -40) -> (66.2, -38.5) centre (66.2, -40) ccw projected
  line L12 (64.7, -40) -> (59.5, -40) projected
  arc A35 (58, -38.5) -> (59.5, -40) centre (58, -40) ccw projected
  line L13 (58, -38.5) -> (58, 0) projected
  line L14 (58, 0) -> (9.2, 0) projected
  line L15 (9.2, 0) -> (9.2, -300) projected
  line L16 (9.2, -300) -> (58, -300) projected
  line L17 (58, -300) -> (58, -261.5) projected
  arc A36 (59.5, -260) -> (58, -261.5) centre (58, -260) ccw projected
  line L18 (59.5, -260) -> (64.7, -260) projected
  arc A37 (66.2, -261.5) -> (64.7, -260) centre (66.2, -260) ccw projected
  line L19 (66.2, -261.5) -> (66.2, -300) projected
  line L20 (66.2, -300) -> (123.8, -300) projected
  line L21 (123.8, -300) -> (123.8, -261.5) projected
  arc A38 (125.3, -260) -> (123.8, -261.5) centre (123.8, -260) ccw projected
  line L22 (125.3, -260) -> (130.5, -260) projected
  arc A39 (132, -261.5) -> (130.5, -260) centre (132, -260) ccw projected
  line L23 (132, -261.5) -> (132, -300) projected
  line L24 (132, -300) -> (180.8, -300) projected
  line L25 (180.8, -300) -> (180.8, 0) projected
  line L26 (180.8, 0) -> (132, 0) projected
  line L27 (132, 0) -> (132, -38.5) projected
  line L28 (9.2, 0) -> (9.2, -300) projected
  circle A40 centre (100, -23) radius 1.5 projected
  line L29 (180.8, -300) -> (180.8, 0) projected
  line L30 (58, -40) -> (58, 0) projected
  circle A41 centre (151.4442, -57.435) radius 1.5 projected
  line L31 (39.5558, -245.9191) -> (39.5558, -298)
  line L32 (134, -298) -> (134, -262.8723)
  line L33 (121.8, -262.8723) -> (121.8, -298)
  line L34 (68.2, -298) -> (68.2, -262.8723)
  line L35 (63.3277, -258) -> (60.8723, -258)
  line L36 (56, -262.8723) -> (56, -298)
  line L37 (138.6723, -215.1) -> (141.1277, -215.1)
  line L38 (146, -210.2277) -> (146, -191.7723)
  line L39 (141.1277, -186.9) -> (138.6723, -186.9)
  line L40 (133.8, -191.7723) -> (133.8, -210.2277)
  line L41 (134, -2) -> (134, -37.1277)
  line L42 (129.1277, -42) -> (126.6723, -42)
  line L43 (121.8, -37.1277) -> (121.8, -2)
  line L44 (68.2, -2) -> (68.2, -37.1277)
  line L45 (56, -2) -> (56, -37.1277)
  line L46 (60.8723, -42) -> (63.3277, -42)
  line L47 (23.1809, -68.4558) -> (11.2, -68.4558)
  line L48 (48.8723, -84.9) -> (51.3277, -84.9)
  line L49 (56.2, -89.7723) -> (56.2, -108.2277)
  line L50 (51.3277, -113.1) -> (48.8723, -113.1)
  line L51 (44, -108.2277) -> (44, -89.7723)
  line L52 (178.8, -298) -> (152.4442, -298)
  line L53 (150.4442, -298) -> (134, -298)
  line L54 (126.6723, -258) -> (129.1277, -258)
  arc A42 (121.8, -37.1277) -> (121.3043, -42.4539) centre (123.8, -40) ccw
  arc A43 (123.0555, -43.4199) -> (126.6723, -42) centre (123.8, -40) ccw
  arc A44 (129.1277, -42) -> (133.8296, -42.9837) centre (132, -40) ccw
  arc A45 (135.1648, -41.4947) -> (134, -37.1277) centre (132, -40) ccw
  line L55 (178.8, -2) -> (152.4442, -2)
  line L56 (150.4442, -2) -> (134, -2)
  line L57 (178.8, -68.4558) -> (178.8, -2)
  line L58 (166.8191, -68.4558) -> (178.8, -68.4558)
  line L59 (166.8191, -70.4558) -> (178.8, -70.4558)
  line L60 (164.465, -72.8099) -> (164.465, -148.5)
  line L61 (162.465, -72.8099) -> (162.465, -148.5)
  arc A46 (164.465, -72.8099) -> (166.8191, -70.4558) centre (163.465, -69.4558) ccw
  arc A47 (166.8191, -68.4558) -> (162.465, -72.8099) centre (163.465, -69.4558) ccw
  line L62 (178.8, -148.5) -> (178.8, -70.4558)
  line L63 (178.8, -148.5) -> (164.465, -148.5)
  arc A48 (155.3495, -148.5) -> (150.4505, -148.5) centre (152.9, -151) ccw
  line L64 (178.8, -151.5) -> (156.3641, -151.5)
  line L65 (162.465, -148.5) -> (155.3495, -148.5)
  arc A49 (149.4359, -151.5) -> (151.1597, -154.0367) centre (152.9, -151) ccw
  arc A50 (153.1067, -154.4939) -> (156.3641, -151.5) centre (152.9, -151) ccw
  line L66 (145.7403, -185.8633) -> (153.1067, -154.4939)
  line L67 (143.7933, -185.4061) -> (151.1597, -154.0367)
  arc A51 (138.6723, -186.9) -> (134.1767, -185.7992) centre (135.8, -188.9) ccw
  arc A52 (132.7437, -187.1944) -> (133.8, -191.7723) centre (135.8, -188.9) ccw
  arc A53 (146, -191.7723) -> (145.7403, -185.8633) centre (144, -188.9) ccw
  arc A54 (143.7933, -185.4061) -> (141.1277, -186.9) centre (144, -188.9) ccw
  arc A55 (133.8, -210.2277) -> (132.3009, -213.1777) centre (135.8, -213.1) ccw
  arc A56 (132.9147, -215.0812) -> (138.6723, -215.1) centre (135.8, -213.1) ccw
  arc A57 (141.1277, -215.1) -> (145.208, -216.3849) centre (144, -213.1) ccw
  arc A58 (146.8097, -215.1871) -> (146, -210.2277) centre (144, -213.1) ccw
  line L68 (146.8097, -215.1871) -> (151.692, -221.7151)
  line L69 (145.208, -216.3849) -> (150.0903, -222.9129)
  line L70 (132.861, -256.6076) -> (150.3218, -227.3671)
  line L71 (134.5782, -257.6329) -> (152.039, -228.3924)
  arc A59 (152.039, -228.3924) -> (151.692, -221.7151) centre (152.9, -225) ccw
  arc A60 (150.0903, -222.9129) -> (150.3218, -227.3671) centre (152.9, -225) ccw
  line L72 (166.8191, -231.5442) -> (178.8, -231.5442)
  line L73 (166.8191, -229.5442) -> (178.8, -229.5442)
  arc A61 (166.8191, -229.5442) -> (160.3862, -232.2088) centre (163.465, -230.5442) ccw
  arc A62 (161.8004, -233.623) -> (166.8191, -231.5442) centre (163.465, -230.5442) ccw
  line L74 (178.8, -298) -> (178.8, -231.5442)
  line L75 (178.8, -229.5442) -> (178.8, -151.5)
  line L76 (152.4442, -245.9191) -> (152.4442, -298)
  line L77 (150.4442, -245.9191) -> (150.4442, -298)
  line L78 (160.3862, -232.2088) -> (153.1088, -239.4862)
  line L79 (161.8004, -233.623) -> (154.523, -240.9004)
  arc A63 (153.1088, -239.4862) -> (150.4442, -245.9191) centre (151.4442, -242.565) ccw
  arc A64 (152.4442, -245.9191) -> (154.523, -240.9004) centre (151.4442, -242.565) ccw
  line L80 (133.7944, -256.995) -> (133.8, -256.9856)
  arc A65 (134, -262.8723) -> (134.5782, -257.6329) centre (132, -260) ccw
  arc A66 (132.861, -256.6076) -> (129.1277, -258) centre (132, -260) ccw
  arc A67 (126.6723, -258) -> (123.0555, -256.5801) centre (123.8, -260) ccw
  arc A68 (121.3043, -257.5461) -> (121.8, -262.8723) centre (123.8, -260) ccw
  line L81 (112.5048, -237.4539) -> (123.0555, -256.5801)
  line L82 (110.7536, -238.4199) -> (121.3043, -257.5461)
  line L83 (96.5, -236) -> (106.655, -236)
  line L84 (96.5, -234) -> (106.655, -234)
  arc A69 (106.655, -236) -> (110.7536, -238.4199) centre (110.0091, -235) ccw
  arc A70 (112.5048, -237.4539) -> (106.655, -234) centre (110.0091, -235) ccw
  line L85 (132.9147, -215.0812) -> (102.3991, -224.9223)
  line L86 (132.3009, -213.1777) -> (101.7853, -223.0188)
  line L87 (96.5, -227.5475) -> (96.5, -234)
  arc A71 (96.5, -227.5475) -> (102.3991, -224.9223) centre (98.9, -225) ccw
  arc A72 (101.7853, -223.0188) -> (96.5, -222.4525) centre (98.9, -225) ccw
  arc A73 (79.2627, -238.4195) -> (83.3632, -236) centre (80.0091, -235) ccw
  arc A74 (83.3632, -234) -> (77.5121, -237.4525) centre (80.0091, -235) ccw
  line L88 (83.3632, -236) -> (93.5, -236)
  line L89 (83.3632, -234) -> (93.5, -234)
  line L90 (79.2627, -238.4195) -> (68.6971, -257.5475)
  line L91 (77.5121, -237.4525) -> (66.9464, -256.5805)
  line L92 (54.8352, -258.5053) -> (40.3855, -245.5487)
  arc A75 (60.8723, -258) -> (56.1704, -257.0163) centre (58, -260) ccw
  arc A76 (54.8352, -258.5053) -> (56, -262.8723) centre (58, -260) ccw
  arc A77 (68.2, -262.8723) -> (68.6971, -257.5475) centre (66.2, -260) ccw
  arc A78 (66.9464, -256.5805) -> (63.3277, -258) centre (66.2, -260) ccw
  line L93 (56.1704, -257.0163) -> (41.7207, -244.0596)
  line L94 (37.5558, -245.9191) -> (37.5558, -298)
  arc A79 (39.5558, -245.9191) -> (40.3855, -245.5487) centre (38.5558, -242.565) ccw
  arc A80 (41.7207, -244.0596) -> (37.5558, -245.9191) centre (38.5558, -242.565) ccw
  line L95 (56, -298) -> (39.5558, -298)
  line L96 (37.5558, -298) -> (11.2, -298)
  line L97 (11.2, -231.5442) -> (11.2, -298)
  line L98 (27.535, -227.1901) -> (27.535, -151.5)
  line L99 (25.535, -227.1901) -> (25.535, -151.5)
  arc A81 (23.1809, -231.5442) -> (27.535, -227.1901) centre (26.535, -230.5442) ccw
  arc A82 (25.535, -227.1901) -> (23.1809, -229.5442) centre (26.535, -230.5442) ccw
  line L100 (23.1809, -231.5442) -> (11.2, -231.5442)
  line L101 (23.1809, -229.5442) -> (11.2, -229.5442)
  line L102 (11.2, -151.5) -> (11.2, -229.5442)
  line L103 (25.535, -151.5) -> (11.2, -151.5)
  line L104 (46, -111.1) -> (45.6571, -112.5603)
  line L105 (33.6359, -148.5) -> (11.2, -148.5)
  line L106 (34.6505, -151.5) -> (27.535, -151.5)
  arc A83 (34.6505, -151.5) -> (39.5495, -151.5) centre (37.1, -149) ccw
  arc A84 (40.5641, -148.5) -> (38.8403, -145.9633) centre (37.1, -149) ccw
  arc A85 (36.8933, -145.5061) -> (33.6359, -148.5) centre (37.1, -149) ccw
  line L107 (54.2, -111.1) -> (55.2464, -112.1747)
  line L108 (87.6359, -148.5) -> (40.5641, -148.5)
  line L109 (88.6505, -151.5) -> (39.5495, -151.5)
  line L110 (93.5, -151.5475) -> (93.5, -234)
  arc A86 (88.0437, -147.2944) -> (87.6359, -148.5) centre (91.1, -149) ccw
  arc A87 (88.6505, -151.5) -> (93.5, -151.5475) centre (91.1, -149) ccw
  arc A88 (93.5, -146.4525) -> (89.4767, -145.8992) centre (91.1, -149) ccw
  line L111 (132.7437, -187.1944) -> (100.5233, -154.1008)
  line L112 (134.1767, -185.7992) -> (101.9563, -152.7056)
  line L113 (149.4359, -151.5) -> (102.3641, -151.5)
  line L114 (150.4505, -148.5) -> (101.3495, -148.5)
  arc A89 (101.3495, -148.5) -> (96.5, -148.4525) centre (98.9, -151) ccw
  arc A90 (96.5, -153.5475) -> (100.5233, -154.1008) centre (98.9, -151) ccw
  arc A91 (101.9563, -152.7056) -> (102.3641, -151.5) centre (98.9, -151) ccw
  line L115 (96.5, -153.5475) -> (96.5, -222.4525)
  arc A92 (56.2, -89.7723) -> (57.6991, -86.8223) centre (54.2, -86.9) ccw
  arc A93 (57.0853, -84.9188) -> (51.3277, -84.9) centre (54.2, -86.9) ccw
  arc A94 (48.8723, -84.9) -> (44.792, -83.6151) centre (46, -86.9) ccw
  arc A95 (43.1903, -84.8129) -> (44, -89.7723) centre (46, -86.9) ccw
  line L116 (54.9165, -110.4024) -> (55.6964, -111.2035)
  line L117 (57.2563, -112.8056) -> (89.4767, -145.8992)
  line L118 (53.4835, -111.7976) -> (54.2634, -112.5987)
  line L119 (55.8233, -114.2008) -> (88.0437, -147.2944)
  line L120 (46.9735, -111.3286) -> (46.7179, -112.417)
  line L121 (46.2067, -114.5939) -> (38.8403, -145.9633)
  line L122 (45.0265, -110.8714) -> (44.7709, -111.9598)
  line L123 (44.2597, -114.1367) -> (36.8933, -145.5061)
  arc A96 (44, -108.2277) -> (44.2597, -114.1367) centre (46, -111.1) ccw
  arc A97 (46.2067, -114.5939) -> (48.8723, -113.1) centre (46, -111.1) ccw
  arc A98 (51.3277, -113.1) -> (55.8233, -114.2008) centre (54.2, -111.1) ccw
  arc A99 (57.2563, -112.8056) -> (56.2, -108.2277) centre (54.2, -111.1) ccw
  line L124 (11.2, -74) -> (33.7459, -74)
  line L125 (11.2, -76) -> (33.7459, -76)
  line L126 (43.1903, -84.8129) -> (38.308, -78.2849)
  line L127 (44.792, -83.6151) -> (39.9097, -77.0871)
  arc A100 (39.9097, -77.0871) -> (39.6782, -72.6329) centre (37.1, -75) ccw
  arc A101 (37.961, -71.6076) -> (33.7459, -74) centre (37.1, -75) ccw
  arc A102 (33.7459, -76) -> (38.308, -78.2849) centre (37.1, -75) ccw
  line L128 (39.6782, -72.6329) -> (57.139, -43.3924)
  line L129 (37.961, -71.6076) -> (55.4218, -42.3671)
  arc A103 (56, -37.1277) -> (55.4218, -42.3671) centre (58, -40) ccw
  arc A104 (57.139, -43.3924) -> (60.8723, -42) centre (58, -40) ccw
  arc A105 (63.3277, -42) -> (66.9464, -43.4195) centre (66.2, -40) ccw
  arc A106 (68.6971, -42.4525) -> (68.2, -37.1277) centre (66.2, -40) ccw
  line L130 (56, -2) -> (39.5558, -2)
  line L131 (37.5558, -2) -> (11.2, -2)
  line L132 (23.1809, -70.4558) -> (11.2, -70.4558)
  line L133 (11.2, -76) -> (11.2, -148.5)
  line L134 (11.2, -2) -> (11.2, -68.4558)
  line L135 (11.2, -70.4558) -> (11.2, -74)
  arc A107 (23.1809, -70.4558) -> (29.6138, -67.7912) centre (26.535, -69.4558) ccw
  arc A108 (28.1996, -66.377) -> (23.1809, -68.4558) centre (26.535, -69.4558) ccw
  arc A109 (36.8912, -60.5138) -> (39.5558, -54.0809) centre (38.5558, -57.435) ccw
  arc A110 (37.5558, -54.0809) -> (35.477, -59.0996) centre (38.5558, -57.435) ccw
  line L136 (39.5558, -54.0809) -> (39.5558, -2)
  line L137 (37.5558, -54.0809) -> (37.5558, -2)
  line L138 (36.8912, -60.5138) -> (29.6138, -67.7912)
  line L139 (35.477, -59.0996) -> (28.1996, -66.377)
  line L140 (91, -19.6459) -> (91, -2)
  line L141 (89, -19.6459) -> (89, -2)
  line L142 (96.6459, -22) -> (93.3541, -22)
  line L143 (99, -2) -> (99, -19.6459)
  line L144 (101, -2) -> (101, -19.6459)
  line L145 (121.8, -2) -> (101, -2)
  arc A111 (99, -19.6459) -> (96.6459, -22) centre (100, -23) ccw
  arc A112 (96.6459, -24) -> (101, -19.6459) centre (100, -23) ccw
  arc A113 (89, -19.6459) -> (93.3541, -24) centre (90, -23) ccw
  arc A114 (93.3541, -22) -> (91, -19.6459) centre (90, -23) ccw
  line L146 (96.6459, -24) -> (96.5, -24)
  line L147 (93.5, -24) -> (93.3541, -24)
  line L148 (93.5, -24) -> (93.5, -64)
  line L149 (96.5, -24) -> (96.5, -64)
  line L150 (96.5, -66) -> (96.5, -148.4525)
  line L151 (93.5, -66) -> (83.3632, -66)
  line L152 (93.5, -64) -> (83.3632, -64)
  line L153 (79.2627, -61.5805) -> (68.6971, -42.4525)
  line L154 (77.5121, -62.5475) -> (66.9464, -43.4195)
  line L155 (106.655, -66) -> (96.5, -66)
  line L156 (106.655, -64) -> (96.5, -64)
  line L157 (121.3043, -42.4539) -> (110.7536, -61.5801)
  line L158 (123.0555, -43.4199) -> (112.5048, -62.5461)
  arc A115 (110.7536, -61.5801) -> (106.655, -64) centre (110.0091, -65) ccw
  arc A116 (106.655, -66) -> (112.5048, -62.5461) centre (110.0091, -65) ccw
  arc A117 (77.5121, -62.5475) -> (83.3632, -66) centre (80.0091, -65) ccw
  arc A118 (83.3632, -64) -> (79.2627, -61.5805) centre (80.0091, -65) ccw
  line L159 (57.0853, -84.9188) -> (87.6009, -75.0777)
  line L160 (57.6991, -86.8223) -> (88.2147, -76.9812)
  line L161 (93.5, -66) -> (93.5, -72.4525)
  line L162 (93.5, -77.5475) -> (93.5, -146.4525)
  arc A119 (93.5, -72.4525) -> (87.6009, -75.0777) centre (91.1, -75) ccw
  arc A120 (88.2147, -76.9812) -> (93.5, -77.5475) centre (91.1, -75) ccw
  line L163 (91, -280.3541) -> (91, -298)
  line L164 (89, -280.3541) -> (89, -298)
  line L165 (96.6459, -278) -> (93.3541, -278)
  line L166 (99, -298) -> (99, -280.3541)
  line L167 (101, -298) -> (101, -280.3541)
  line L168 (96.5, -236) -> (96.5, -276)
  arc A121 (101, -280.3541) -> (96.6459, -276) centre (100, -277) ccw
  arc A122 (96.6459, -278) -> (99, -280.3541) centre (100, -277) ccw
  line L169 (93.5, -236) -> (93.5, -276)
  line L170 (96.6459, -276) -> (96.5, -276)
  line L171 (93.5, -276) -> (93.3541, -276)
  arc A123 (93.3541, -276) -> (89, -280.3541) centre (90, -277) ccw